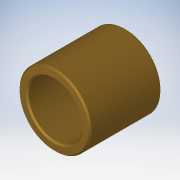
# Autodesk Inventor part: Brass Bushing
Saved by Autodesk Inventor 2018.2 (Build 222227000, 227)
## iProperties
Created: 2018-02-12
Part Number: Brass Bushing
Material: Brass, Soft Yellow
Document SubType Name: Modeling
Designer: Moochster
Density: 8.47 g/cm^3
Appearance: Brass - Satin
Author: Moochster
Autodesk Inventor part; units mm, degrees
ref_plane "YZ Plane" through (0, 0, 0) normal (1, 0, 0) x (0, 1, 0)
ref_plane "XZ Plane" through (0, 0, 0) normal (0, 1, 0) x (-1, 0, 0)
ref_plane "XY Plane" through (0, 0, 0) normal (0, 0, 1) x (1, 0, 0)
sketch "Sketch1" plane through (0, 0, 0) normal (0, 1, 0) x (-1, 0, 0)
  circle A0 centre (0, 0) radius 6.35
  circle A1 centre (0, 0) radius 4.7625
  dimension "d0" = 12.7
  dimension "d1" = 9.525
  constraints: 2 centre point, 2 coincident
  measures "d0" diameter of A0
  measures "d1" diameter of A1
extrude "Extrusion1" add sketch "Sketch1" along normal blind 12.7
chamfer "Chamfer1" distance 0.25 angle 45 4 edges at (6.35, 0, 0) (4.7625, 0, 0) (6.35, 12.7, 0) (4.7625, 12.7, 0)
body "Solid1"
